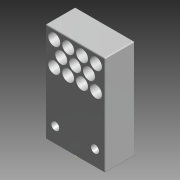
# Autodesk Inventor part: Schlauchhalter
Saved by Autodesk Inventor 2013 (Build 170138000, 138)
## iProperties
Created: 2012-07-25
Part Number: Schlauchhalter
Material: Allgemein
Document SubType Name: Modeling
Designer: fivef
Density: 1 g/cm^3
Mass: 17.3586 g
Surface Area: 81.1341 cm^2
Volume: 17.3586 cm^3
Author: fivef
Autodesk Inventor part; units mm, degrees
ref_plane "YZ Plane" through (0, 0, 0) normal (1, 0, 0) x (0, 1, 0)
ref_plane "XZ Plane" through (0, 0, 0) normal (0, 1, 0) x (-1, 0, 0)
ref_plane "XY Plane" through (0, 0, 0) normal (0, 0, 1) x (1, 0, 0)
sketch "Skizze1" plane through (0, 0, 0) normal (0, 1, 0) x (-1, 0, 0)
  line L0 (-24.6188, -3.2813) -> (5.3812, -3.2813)
  line L1 (5.3812, -3.2813) -> (5.3812, 46.7188)
  line L2 (5.3812, 46.7188) -> (-24.6188, 46.7188)
  line L3 (-24.6188, 46.7188) -> (-24.6188, -3.2813)
  line L4 (-24.6188, -3.2813) -> (5.3812, 46.7188) construction
  line L5 (5.3812, -3.2813) -> (-24.6188, 46.7188) construction
  point P0 (0, 0)
  point P1 (-9.6188, 21.7188)
  dimension "d5" = 50
  dimension "d7" = 30
  constraints: 12 end point, 2 midpoint, 2 parallel, 1 horizontal, 1 perpendicular
  measures "d5" distance of L0.end L1.end
  measures "d7" distance of L0.start L0.end
extrude "Extrusion1" add sketch "Skizze1" along normal blind 15
fillet "Rundung1" radius 0.5 12 edges at (24.6188, 7.5, 46.7188) (24.6188, 7.5, -3.2813) (24.6188, 0, 21.7188) (24.6188, 15, 21.7188) (-5.3812, 7.5, 46.7188) (9.6188, 0, 46.7188) (9.6188, 15, 46.7188) (-5.3812, 7.5, -3.2813) (-5.3812, 0, 21.7187) (-5.3812, 15, 21.7187) (9.6188, 0, -3.2813) (9.6188, 15, -3.2813)
sketch "Skizze2" plane through (-4.8812, 15, -2.7813) normal (0, 1, 0) x (1, 0, 0)
  line L0 (29, -49) -> (0, -49) projected
  circle A0 centre (25, -45) radius 3
  circle A1 centre (21.5, -38.9378) radius 3
  line L1 (29.5, -49) -> (29.5, 0) construction
  line L2 (0, -49.5) -> (29, -49.5) construction
  circle A2 centre (18, -45) radius 3
  circle A3 centre (11, -45) radius 3
  circle A4 centre (4, -45) radius 3
  circle A5 centre (25, -32.8756) radius 3
  circle A6 centre (14.5, -38.9378) radius 3
  circle A7 centre (7.5, -38.9378) radius 3
  circle A8 centre (18, -32.8756) radius 3
  circle A9 centre (11, -32.8756) radius 3
  circle A10 centre (4, -32.8756) radius 3
  point P0 (4.8812, -2.7813)
  dimension "d9" = 6
  dimension "d66" = 7
  dimension "d81" = 4.5
  dimension "d82" = 4.5
  dimension "d86" = 7
  dimension "d93" = 7
  dimension "d112" = 0
  dimension "d113" = 1
  dimension "d115" = 1
  dimension "d116" = 1
  dimension "d117" = 6.0622
  constraints: 11 centre point, 3 horizontal, 2 equal radius, 16 other
  measures "d9" diameter of A0
  measures "d66" distance of A0.centre A2.centre
  measures "d81" distance from line of L1 A0.centre
  measures "d82" distance from line of A0.centre L2
  measures "d86" distance of A1.centre A6.centre
  measures "d93" distance of A5.centre A8.centre
  measures "d112" horizontal distance of A0.centre A5.centre
  measures "d117" vertical distance of A1.centre A5.centre
extrude "Extrusion2" cut sketch "Skizze2" against normal through all
sketch "Skizze3" plane through (0, 15, 0) normal (0, 1, 0) x (1, 0, 0)
  circle A0 centre (-0.3812, -4.7187) radius 2
  circle A1 centre (19.6188, -4.7187) radius 2
  line L0 (24.1188, 3.2813) -> (-4.8812, 3.2813) projected
  line L1 (24.6188, -46.2187) -> (24.6188, 2.7813) projected
  line L2 (-5.3812, 2.7813) -> (-5.3812, -46.2188) projected
  point P0 (0, 0)
  dimension "d40" = 4
  dimension "d43" = 4
  dimension "d105" = 8
  dimension "d106" = 8
  dimension "d107" = 5
  dimension "d108" = 5
  dimension "d118" = 20
  constraints: 2 centre point
  measures "d40" diameter of A0
  measures "d43" diameter of A1
  measures "d105" distance from line of L0 A0.centre
  measures "d106" distance from line of A1.centre L0
  measures "d107" distance from line of L1 A1.centre
  measures "d108" distance from line of L2 A0.centre
  measures "d118" distance of A1.centre A0.centre
hole "Bohrung1" at (-0.3812, 15, 4.7187) at (19.6188, 15, 4.7187) direction (0, -1, 0) diameter 4 end through all countersink diameter 8.3 countersink angle 90
